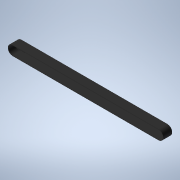
# Autodesk Inventor part: HTBN360S2M-100_info-1-16-16
Saved by Autodesk Inventor 2021 (Build 250183000, 183)
## iProperties
Created: 2025-03-04
Part Number: HTBN360S2M-100_info-1-16-16
Material: Generic
Catalog Web Link: www.cadenas.de
Description: HTBN_ _S2M, HTUN_ _S2M-High Torque Timing Belts S2M (Pitch 2mm)
Vendor: MISUMI
Document SubType Name: Modeling
Designer: psAdmin
Manufacturer: MISUMI
Mass: 2.20518 g
Surface Area: 77.0346 cm^2
Volume: 2.20518 cm^3
Density: 1 g/cm^3
Appearance: PSOLRGB-175-175-175
Category: PARTsolutions
Company: MISUMI
Title: HTBN360S2M-100
Author: Cadenas PARTsolutions
Comments: High Torque Timing Belts S2M (Pitch 2mm)
PSOL_IDENT_0: {$CADENAS_DATA/23d-libs/misumi/metric/48_timing_belts/htbn_s2m.prj},225 {VTYP=3D},{NB=HTBN360S2M-100
PSOL_IDENT_1: _info-1-16-16},{LINA=HTBN360S2M-100},{NN=HTBN_ _S2M, HTUN_ _S2M},{DATE=17.01.2023 06:33:33},{GEOMDAT
PSOL_IDENT_2: E=05.10.2021 14:18:16},{VERSION=},{LINEID=40},{WBVAR=TS,NT,RSSP,NT1,NT2},{WBNUMERIC=NT,NT1,NT2}  {NB=
PSOL_IDENT_3: HTBN360S2M-100_info-1-16-16},{LINA=HTBN360S2M-100},{KT=DUMMY},{PN=HTBN360S2M-100},{TS=HTBN},{MATBR=C
PSOL_IDENT_4: hloroprene Rubber},{MATTR=Chloroprene Rubber},{MATCW=Glass Fiber Cord},{MATBC=Nylon Cloth},{OT=-30~9
PSOL_IDENT_5: 0},{BNO=360S2M},{BNW=10},{NT=180},{BC=360},{PITCH=2},{RAA=1.3},{LRR=1.3},{H=1.36},{HH=0.76},{II=0.6}
PSOL_IDENT_6: ,{PLD=0.254},{BNWALG=100},{NTALG=33,38,39,40,44,45,50,56,58,59,61,62,63,64,65,66,67,69,70,71,72,76,8
PSOL_IDENT_7: 0,82,83,86,88,90,93,95,97,100,102,105,106,107,110,112,115,117,118,122,123,125,128,133,140,145,150,16
PSOL_IDENT_8: 0,162,164,165,170,180,185,190,200,218,224,250,260,280,300,315,355,400,450,492,598,625,637,645,710,75
PSOL_IDENT_9: 8,762,939,1065},{RSSP=1},{RSSP1= '1','900 or Less','2','Over 900, 1200 or Less','3','Over 1200, 1800
PSOL_IDENT_10: or Less','4','Over 1800, 3600 or Less','5','Over 3600, 4800 or Less','6','Over 4800, 10000 or Less'
PSOL_IDENT_11: },{NT1=16},{NT2=16},{NT1A=16,18,20,22,23,24,25,26,28,30,32,34,36,40,44,48,50,60},{NT1A0=0},{NT1A1=1
PSOL_IDENT_12: 6,18,20,22,23,24,25,26,28,30,32,34,36,40,44,48,50,60},{NT2A=16,18,20,22,23,24,25,26,28,30,32,34,36,4
PSOL_IDENT_13: 0,44,48,50,60,72},{DRIVEP=10.18592},{DRIVENP=10.18592},{DRP=9.677916},{DRNP=9.677916},{DRP1=9.680},{
PSOL_IDENT_14: DRNP1=9.680},{C=164.00},{BB=656.00000},{NOTE=-},{ASSCFGC=NT2,C},{ASSCFGCNOTE=-},{FS=14.00},{FL=14.00
PSOL_IDENT_15: },{NT1SCR=16,18,20,22,23,24,25,26,28,30,32,34,36,40,44,48,50,60},{NT2SCR=16,18,20,22,23,24,25,26,28,
PSOL_IDENT_16: 30,32,34,36,40,44,48,50,60,72}
NB: HTBN360S2M-100_info-1-16-16
NN: HTBN_ _S2M, HTUN_ _S2M
NT: 180
NBSYN: $PN._info-$RSSP.-$NT1.-$NT2.
LINA: HTBN360S2M-100
CATALOG: Misumi
PN: HTBN360S2M-100
TS: Rubber
MATBR: Chloroprene Rubber
MATTR: Chloroprene Rubber
MATCW: Glass Fiber Cord
MATBC: Nylon Cloth
OT: -30~90
BNO: 360S2M
BNW: 10
BC: 360
PITCH: 2
RAA: 1.3
LRR: 1.3
H: 1.36
HH: 0.76
II: 0.6
PLD: 0.254
RSSP: 900 or Less
NT1: 16
NT2: 16
C: 164
NOTE: -
SUPPLIER: MISUMI
ARTICLENO: HTBN360S2M-100_info-1-16-16
BOMINFO: HTBN360S2M-100
CREATOR: CADENAS GmbH
Autodesk Inventor part; units mm, degrees
ref_plane "YZ Plane" through (0, 0, 0) normal (1, 0, 0) x (0, 1, 0)
ref_plane "XZ Plane" through (0, 0, 0) normal (0, 1, 0) x (-1, 0, 0)
ref_plane "XY Plane" through (0, 0, 0) normal (0, 0, 1) x (1, 0, 0)
sketch "Sketch_1" plane through (0, 0, 0) normal (0, 0, 1) x (1, 0, 0)
  line L0 (4, 4.839) -> (4.35, 4.839)
  arc A0 (4.35, 4.839) -> (4.5953, 4.079) centre (5.65, 4.839) ccw
  line L1 (4.5953, 4.079) -> (5.4047, 4.079)
  arc A1 (5.4047, 4.079) -> (5.65, 4.839) centre (4.35, 4.839) ccw
  line L2 (5.65, 4.839) -> (6.35, 4.839)
  arc A2 (6.35, 4.839) -> (6.5953, 4.079) centre (7.65, 4.839) ccw
  line L3 (6.5953, 4.079) -> (7.4047, 4.079)
  arc A3 (7.4047, 4.079) -> (7.65, 4.839) centre (6.35, 4.839) ccw
  line L4 (7.65, 4.839) -> (8.35, 4.839)
  arc A4 (8.35, 4.839) -> (8.5953, 4.079) centre (9.65, 4.839) ccw
  line L5 (8.5953, 4.079) -> (9.4047, 4.079)
  arc A5 (9.4047, 4.079) -> (9.65, 4.839) centre (8.35, 4.839) ccw
  line L6 (9.65, 4.839) -> (10.35, 4.839)
  arc A6 (10.35, 4.839) -> (10.5953, 4.079) centre (11.65, 4.839) ccw
  line L7 (10.5953, 4.079) -> (11.4047, 4.079)
  arc A7 (11.4047, 4.079) -> (11.65, 4.839) centre (10.35, 4.839) ccw
  line L8 (11.65, 4.839) -> (12.35, 4.839)
  arc A8 (12.35, 4.839) -> (12.5953, 4.079) centre (13.65, 4.839) ccw
  line L9 (12.5953, 4.079) -> (13.4047, 4.079)
  arc A9 (13.4047, 4.079) -> (13.65, 4.839) centre (12.35, 4.839) ccw
  line L10 (13.65, 4.839) -> (14, 4.839)
  line L11 (14, 4.839) -> (14, 5.439)
  line L12 (14, 5.439) -> (4, 5.439)
  line L13 (4, 5.439) -> (4, 4.839)
  constraints: 28 end point, 20 point on circle, 10 centre point
extrude "Extrusion1" add sketch "Sketch_1" along normal mid plane 10
sketch "Sketch_3" plane through (0, 0, 0) normal (0, 0, 1) x (1, 0, 0)
  arc A0 (0, 5.439) -> (0, -5.439) centre (0, 0) ccw
  line L0 (0, -5.439) -> (164, -5.439)
  arc A1 (164, -5.439) -> (164, 5.439) centre (164, 0) ccw
  line L1 (164, 5.439) -> (0, 5.439)
  arc A2 (0, 4.839) -> (0, -4.839) centre (0, 0) ccw
  line L2 (0, -4.839) -> (164, -4.839)
  arc A3 (164, -4.839) -> (164, 4.839) centre (164, 0) ccw
  line L3 (164, 4.839) -> (0, 4.839)
  constraints: 8 end point, 8 point on circle, 4 centre point
extrude "Extrusion2" add sketch "Sketch_3" along normal mid plane 10
ref_plane "C1_XY" through (0, 0, 0) normal (0, 0, 1) x (1, 0, 0)
ref_plane "C1_YZ" through (0, 0, 0) normal (1, 0, 0) x (0, 1, 0)
ref_plane "C1_ZX" through (0, 0, 0) normal (0, 1, 0) x (0, 0, 1)
ref_plane "C2_XY" through (164, 0, 0) normal (0, 0, 1) x (1, 0, 0)
ref_plane "C2_YZ" through (164, 0, 0) normal (1, 0, 0) x (0, 1, 0)
ref_plane "C2_ZX" through (164, 0, 0) normal (0, 1, 0) x (0, 0, 1)
body "Solid1"
